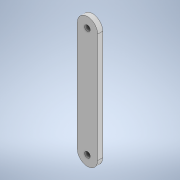
# Autodesk Inventor part: Eslabon
Saved by Autodesk Inventor 2022 (Build 260153000, 153)
## iProperties
Created: 2022-01-10
Part Number: Eslabon
Material: Generic
Document SubType Name: Modeling
Designer: Yeison
Density: 1 g/cm^3
Appearance: Default
Author: Yeison
Autodesk Inventor part; units mm, degrees
ref_plane "YZ Plane" through (0, 0, 0) normal (1, 0, 0) x (0, 1, 0)
ref_plane "XZ Plane" through (0, 0, 0) normal (0, 1, 0) x (-1, 0, 0)
ref_plane "XY Plane" through (0, 0, 0) normal (0, 0, 1) x (1, 0, 0)
sketch "Sketch4" plane through (0, 0, 0) normal (0, 0, 1) x (1, 0, 0)
  line L0 (20, -107.5) -> (20, 107.5)
  line L1 (-20, 107.5) -> (-20, -107.5)
  line L2 (-20, -107.5) -> (20, 107.5) construction
  line L3 (20, -107.5) -> (-20, 107.5) construction
  circle A0 centre (0, 107.5) radius 5.5
  arc A1 (20, 107.5) -> (-20, 107.5) centre (0, 107.5) ccw
  circle A2 centre (0, -107.5) radius 5.5
  arc A3 (-20, -107.5) -> (20, -107.5) centre (0, -107.5) ccw
  point P0 (0, 0)
  dimension "d20" = 40
  dimension "d21" = 215
  dimension "d22" = 11
  dimension "d23" = 11
  constraints: 8 end point, 4 centre point, 4 point on circle, 2 coincident, 2 midpoint, 1 parallel
  measures "d20" distance of L1.start L0.end
  measures "d21" distance of L0.start L0.end
  measures "d22" diameter of A0
  measures "d23" diameter of A2
extrude "Extrusion3" add sketch "Sketch4" along normal blind 10
body "Solid3"
